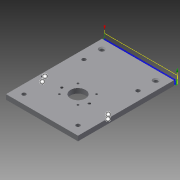
# Autodesk Inventor part: motor plate support
Saved by Autodesk Inventor 2015 SP1 (Build 190203100, 203)
## iProperties
Created: 2015-04-23
Part Number: motor plate support
Material: Generic
Document SubType Name: Modeling
Designer: ubik
Density: 1 g/cm^3
Appearance: Default
Mass: 147.269 g
Surface Area: 436.578 cm^2
Volume: 147.269 cm^3
Author: ubik
Autodesk Inventor part; units mm, degrees
ref_plane "YZ Plane" through (0, 0, 0) normal (1, 0, 0) x (0, 1, 0)
ref_plane "XZ Plane" through (0, 0, 0) normal (0, 1, 0) x (-1, 0, 0)
ref_plane "XY Plane" through (0, 0, 0) normal (0, 0, 1) x (1, 0, 0)
sketch "Sketch1" plane through (0, 0, 0) normal (0, 0, 1) x (1, 0, 0)
  line L0 (0, 0) -> (120, 0)
  line L1 (120, 0) -> (120, 160)
  line L2 (120, 160) -> (0, 160)
  line L3 (0, 160) -> (0, 0)
  dimension "width" = 120
  dimension "d1" = 160
  constraints: 8 end point, 2 parallel, 1 horizontal, 1 perpendicular
  measures "width" distance of L2.end L1.end
  measures "d1" distance of L1.end L0.end
extrude "Extrusion1" add sketch "Sketch1" along normal blind 8
hole "Hole1" at (15, 15, 8) direction (0, 0, -1) diameter 6.5 end through all
pattern_linear "Rectangular Pattern1" count 2 spacing 90 along (1, 0, 0) count 2 spacing 100 along (0, 1, 0) of "Hole1"
hole "Hole2" at (15, 145, 8) direction (0, 0, -1) diameter 6.5 end through all countersink diameter 10 countersink angle 90
pattern_linear "Rectangular Pattern2" count 2 spacing 90 along (1, 0, 0) of "Hole2"
hole "Hole3" at (60, 60, 8) direction (0, 0, -1) diameter 25 end through all
hole "Hole4" at (44.5, 75.5, 8) direction (0, 0, -1) diameter 3.5 end through all
pattern_linear "Rectangular Pattern3" count 2 spacing 31 along (0, -1, 0) count 2 spacing 31 along (1, 0, 0) of "Hole4"
hole "Hole5" at (5, 56, 8) direction (0, 0, -1) diameter 4.134 end through all thread size "M5x0.8" class "6H" standard "ANSI Metric M Profile"
hole "Hole6" at (115, 56, 8) direction (0, 0, -1) diameter 4.134 end through all thread size "M5x0.8" class "6H" standard "ANSI Metric M Profile"
pattern_linear "Rectangular Pattern4" count 2 spacing 32 along (1, 0, 0) of "Hole5"
pattern_linear "Rectangular Pattern5" count 2 spacing 32 along (-1, 0, 0) of "Hole6"
body "Solid1"
